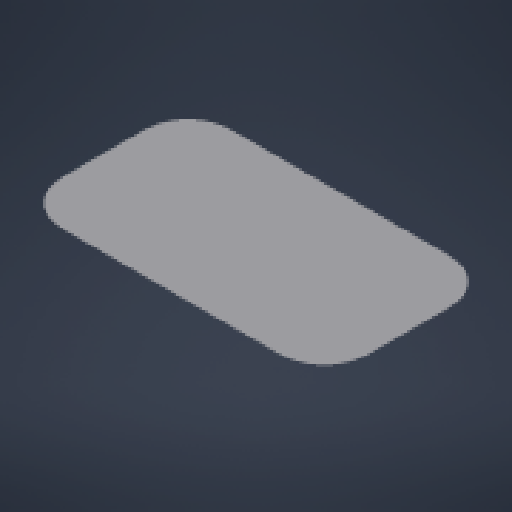
# Autodesk Inventor part: Base
Saved by Autodesk Inventor 2026.1 (Build 301233000, 233)
## iProperties
Manager: MANUTENÇÃO GUIFÕES - CP
Company: CP
Created: 2025-09-03
Part Number: Base
Project: 0.00 0000/00
Checked By: PMFIGUEIREDO
Engr Approved By: JSSILVA
Material: Generic
Description: NOME DA PEÇA
Document SubType Name: Modeling
Designer: TPMIRANDA
Engineer: ISO 2768 - m K
Authority: Nº DESENHO PELO QUAL FOI SUBSITUIDO
Stock Number: 00000-000
Density: 1 g/cm^3
Appearance: Default
Title: UME 3400
Subject: CAIXA, INTERIOR, SUPORTE,
Author: TPMIRANDA
Keywords: Caixa de comentários. Substituir texto, ou eliminar.
Comments: UQE2300 UQE2400 UTE2240 UDD9630 CARRUAGENS SIMAFE CARRUAGENS CAF CARRUAGENS ARCO
Revision Number: Nº DESENHO QUE SUBSTITUI
Autodesk Inventor part; units mm, degrees
ref_plane "YZ Plane" through (0, 0, 0) normal (1, 0, 0) x (0, 1, 0)
ref_plane "XZ Plane" through (0, 0, 0) normal (0, 1, 0) x (-1, 0, 0)
ref_plane "XY Plane" through (0, 0, 0) normal (0, 0, 1) x (1, 0, 0)
sketch "Sketch1" plane through (0, 0, 0) normal (0, 0, 1) x (1, 0, 0)
  line L0 (-4.5, -2.5) -> (4.5, -2.5)
  line L1 (4.5, -2.5) -> (4.5, 2.5)
  line L2 (4.5, 2.5) -> (-4.5, 2.5)
  line L3 (-4.5, 2.5) -> (-4.5, -2.5)
  line L4 (-4.5, -2.5) -> (4.5, 2.5) construction
  line L5 (4.5, -2.5) -> (-4.5, 2.5) construction
  point P0 (0, 0)
  dimension "d0" = 9
  dimension "d1" = 5
  constraints: 12 end point, 2 midpoint, 2 parallel, 1 horizontal, 1 perpendicular
  measures "d0" distance of L1.end L2.end
  measures "d1" distance of L2.end L0.start
extrude "Extrusion1" add sketch "Sketch1" against normal blind 0.7 draft -45
fillet "Fillet1" radius 2 4 edges at (-4.15, -2.15, -0.35) (-4.15, 2.15, -0.35) (4.15, -2.15, -0.35) (4.15, 2.15, -0.35)
body "Solid1"
